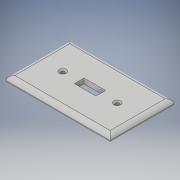
# Autodesk Inventor part: Plate
Saved by Autodesk Inventor 2019 (Build 230136000, 136)
## iProperties
Created: 2019-02-03
Part Number: Plate
Material: Generic
Document SubType Name: Modeling
Designer: Jared
Density: 1 g/cm^3
Appearance: Default
Author: Jared
Autodesk Inventor part; units mm, degrees
ref_plane "YZ Plane" through (0, 0, 0) normal (1, 0, 0) x (0, 1, 0)
ref_plane "XZ Plane" through (0, 0, 0) normal (0, 1, 0) x (-1, 0, 0)
ref_plane "XY Plane" through (0, 0, 0) normal (0, 0, 1) x (1, 0, 0)
sketch "Sketch1" plane through (0, 0, 0) normal (0, 1, 0) x (-1, 0, 0)
  line L0 (-56.75, -34.75) -> (56.75, -34.75)
  line L1 (56.75, -34.75) -> (56.75, 34.75)
  line L2 (56.75, 34.75) -> (-56.75, 34.75)
  line L3 (-56.75, 34.75) -> (-56.75, -34.75)
  line L4 (-56.75, -34.75) -> (56.75, 34.75) construction
  line L5 (56.75, -34.75) -> (-56.75, 34.75) construction
  point P0 (0, 0)
  dimension "d0" = 113.5
  dimension "d1" = 69.5
  constraints: 12 end point, 2 midpoint, 2 parallel, 1 horizontal, 1 perpendicular
  measures "d0" distance of L2.end L1.end
  measures "d1" distance of L1.end L0.end
extrude "Extrusion1" add sketch "Sketch1" along normal blind 5.5
sketch "Sketch2" plane through (0, 5.5, 0) normal (0, 1, 0) x (1, 0, 0)
  line L0 (56.75, 34.75) -> (-56.75, 34.75) projected
  line L1 (-56.75, 34.75) -> (-56.75, -34.75) projected
  line L2 (-56.75, -34.75) -> (56.75, -34.75) projected
  line L3 (56.75, -34.75) -> (56.75, 34.75) projected
  line L4 (11.75, -5.25) -> (-11.75, -5.25)
  line L5 (-11.75, -5.25) -> (-11.75, 5.25)
  line L6 (-11.75, 5.25) -> (11.75, 5.25)
  line L7 (11.75, 5.25) -> (11.75, -5.25)
  line L8 (11.75, -5.25) -> (-11.75, 5.25) construction
  line L9 (-11.75, -5.25) -> (11.75, 5.25) construction
  point P0 (0, 0)
  dimension "d4" = 45
  dimension "d5" = 29.5
  constraints: 12 end point, 2 midpoint, 2 parallel, 1 horizontal, 1 perpendicular
  measures "d4" distance between parallel lines of L3 L7
  measures "d5" distance between parallel lines of L0 L6
extrude "Extrusion2" cut sketch "Sketch2" against normal up to next contours L4 L5 L6 L7
sketch "Sketch3" plane through (0, 5.5, 0) normal (0, 1, 0) x (1, 0, 0)
  line L0 (11.75, 5.25) -> (11.75, -5.25) projected
  line L1 (11.75, 0) -> (29.75, 0)
  line L2 (-11.75, 5.25) -> (-11.75, -5.25) projected
  line L3 (-11.75, 0) -> (-29.75, 0)
  point P0 (0, 0)
  dimension "d8" = 18
  constraints: 4 end point, 2 coincident, 2 horizontal, 2 midpoint, 1 collinear
  measures "d8" distance of L1.start L1.end
hole "Hole1" at (-29.75, 5.5, 0) at (29.75, 5.5, 0) direction (0, -1, 0) diameter 4.5 depth 10 tip angle 118 countersink diameter 7.5 countersink angle 90
fillet "Fillet1" radius 4.75 4 edges at (-56.75, 5.5, 0) (56.75, 5.5, 0) (0, 5.5, 34.75) (0, 5.5, -34.75)
body "Solid1"
